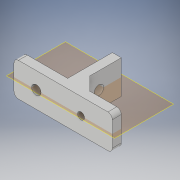
# Autodesk Inventor part: HeatbedMount
Saved by Autodesk Inventor 2018 (Build 220112000, 112)
## iProperties
Created: 2017-10-07
Part Number: HeatbedMount
Material: Generic
Document SubType Name: Modeling
Designer: Jurjen
Density: 1 g/cm^3
Appearance: Default
Author: Jurjen
Autodesk Inventor part; units mm, degrees
ref_plane "YZ Plane" through (0, 0, 0) normal (1, 0, 0) x (0, 1, 0)
ref_plane "XY Plane" through (0, 0, 0) normal (0, 0, 1) x (1, 0, 0)
sketch "Sketch1" plane through (0, 0, 0) normal (0, 1, 0) x (-1, 0, 0)
  line L0 (22, 14) -> (-22, 14)
  line L1 (-22, 14) -> (-22, 10)
  line L2 (-22, 10) -> (-2, 10)
  line L3 (-2, 10) -> (-2, -10)
  line L4 (-2, -10) -> (2, -10)
  line L5 (2, -10) -> (2, 10)
  line L6 (2, 10) -> (22, 10)
  line L7 (22, 10) -> (22, 14)
  point P0 (0, 0)
  point P1 (-2, 0)
  point P2 (0, 14)
  dimension "d0" = 20
  dimension "d1" = 4
  dimension "d2" = 20
  dimension "d3" = 4
  dimension "d4" = 20
  constraints: 16 end point, 7 perpendicular, 2 horizontal alignment, 2 midpoint, 1 horizontal, 1 vertical alignment
  measures "d0" distance of L5.end L6.end
  measures "d1" distance between parallel lines of L3 L5
  measures "d2" distance between parallel lines of L4 L6
  measures "d3" distance of L6.end L0.start
  measures "d4" distance of L1.end L2.end
extrude "Extrusion1" add sketch "Sketch1" along normal mid plane 15
sketch "Sketch2" plane through (-2, -7.5, 10) normal (0, 0, -1) x (-1, 0, 0)
  line L0 (20, 0) -> (0, 0) projected
  line L1 (20, 0) -> (20, 15) projected
  line L2 (0, 15) -> (20, 15) projected
  line L3 (0, 0) -> (0, 15) projected
  circle A0 centre (10, 7.5) radius 2.1
  point P0 (-2, 7.5)
  point P1 (20, 7.5)
  point P2 (10, 0)
  dimension "d7" = 4.2
  constraints: 2 midpoint, 1 centre point, 1 horizontal alignment, 1 vertical alignment
  measures "d7" diameter of A0
extrude "Extrusion2" cut sketch "Sketch2" against normal up to next contours A0
sketch "Sketch3" plane through (2, -7.5, 10) normal (1, 0, 0) x (0, 0, -1)
  line L0 (20, 0) -> (0, 0) projected
  line L1 (20, 0) -> (20, 15) projected
  line L2 (0, 15) -> (20, 15) projected
  line L3 (0, 0) -> (0, 15) projected
  circle A0 centre (10, 7.5) radius 2.1
  point P0 (20, 7.5)
  point P1 (10, 0)
  dimension "d10" = 4.2
  constraints: 2 midpoint, 1 centre point, 1 horizontal alignment, 1 vertical alignment
  measures "d10" diameter of A0
extrude "Extrusion3" cut sketch "Sketch3" against normal up to next contours A0
sketch "Sketch4" plane through (22, -7.5, 10) normal (0, 0, -1) x (-1, 0, 0)
  circle A0 centre (14, 7.5) radius 1.55
  line L0 (0, 0) -> (0, 15) projected
  point P0 (22, 7.5)
  point P1 (0, 7.5)
  dimension "d13" = 3.1
  dimension "d14" = 14
  constraints: 1 centre point, 1 horizontal alignment, 1 midpoint
  measures "d13" diameter of A0
  measures "d14" distance of point (0, 7.5) A0.centre
extrude "Extrusion4" cut sketch "Sketch4" against normal up to next
sketch "Sketch5" plane through (0, 7.5, 0) normal (0, 1, 0) x (1, 0, 0)
  line L0 (2, -4) -> (8, -10)
  line L1 (22, -10) -> (2, -10) projected
  line L2 (2, -10) -> (2, -4)
  line L3 (8, -10) -> (2, -10)
  point P0 (0, 0)
  dimension "d17" = 6
  dimension "d18" = 6
  constraints: 6 end point, 1 collinear, 1 perpendicular, 1 point on line
  measures "d17" distance of L1.end L0.start
  measures "d18" distance of L1.end L0.end
extrude "Extrusion5" add sketch "Sketch5" against normal blind 3
mirror "Mirror1" about plane through (0, 0, 0) normal (0, 1, 0) of "Extrusion5"
fillet "Fillet1" radius 2 4 edges at (-22, 7.5, 12) (22, 7.5, 12) (22, -7.5, 12) (-22, -7.5, 12)
body "Solid1"
